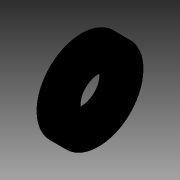
# Autodesk Inventor part: 2281_p2
Saved by Autodesk Inventor 2014 SP2 (Build 180246200, 246)
## iProperties
Created: 2019-11-08
Part Number: 2281_p2
Material: Generic
Catalog Web Link: www.cadenas.de
Description: 2281, 2282, 2280, 2290_p2-Roller Wheels
Vendor: 8020
Document SubType Name: Modeling
Designer: psadmin
Manufacturer: 8020
Mass: 0.492643 g
Surface Area: 5.37288 cm^2
Volume: 0.492643 cm^3
Density: 1 g/cm^3
Appearance: PSOLRGB-0-0-0
Category: PARTsolutions
Company: 8020
Title: 2281_p2
Author: Cadenas PARTsolutions
Comments: Roller Wheels
PSOL_IDENT_0: {$CADENAS_DATA\23d-libs\8020\inch\linear_motion\2281_p2.prj},178 {VTYP=3D},{NB=2281_p2},{LINA=2281_p
PSOL_IDENT_1: 2},{NN=2281, 2282, 2280, 2290_p2},{DATE=01.10.2019 06:04:24},{GEOMDATE=20.12.2011 00:00:00},{VERSION=
PSOL_IDENT_2: },{LINEID=10},{WBVAR=BT,RI},{WBNUMERIC=}  {NB=2281_p2},{LINA=2281_p2},{KT=DUMMY},{PN=2281},{NO=1},{M
PSOL_IDENT_3: AT=Self-lubricating, fiberglass-reinforced black nylon.},{BT=2},{BT1= '2','Permanent Lubricated Bron
PSOL_IDENT_4: ze Bushing' },{MT=10 Series},{RI=10},{RI1= '10','10 Series','15','15 Series' },{A=1.500},{B=1.125},{
PSOL_IDENT_5: C=0.240},{D=0.480},{E=0.563},{F=0.188},{G=0.314},{H=0.214},{J=0.118},{K=0.622},{L=0.429},{M=0.320},{
PSOL_IDENT_6: N=1/4-20},{N1=0.2500},{P=0.060},{Q=0.378},{W=.070},{G1=0.375},{K1=0.000}
NN: 2281, 2282, 2280, 2290_p2
NT: Roller Wheels
NB: 2281_p2
NBSYN: $PN._p2
LINA: 2281_p2
PN: 2281
MAT: Self-lubricating, fiberglass-reinforced black nylon.
BT: Permanent Lubricated Bronze Bushing
MT: 10 Series
RI: 10 Series
A: 1.5
B: 1.125
C: 0.24
D: 0.48
E: 0.563
F: 0.188
G: 0.314
H: 0.214
J: 0.118
K: 0.622
L: 0.429
M: 0.32
N: 1/4-20
P: 0.06
Q: 0.378
W: .070
SUPPLIER: 8020
ARTICLENO: 2281_p2
BOMINFO: 2281_p2
CREATOR: CADENAS GmbH
Autodesk Inventor part; units mm, degrees
ref_plane "YZ Plane" through (0, 0, 0) normal (1, 0, 0) x (0, 1, 0)
ref_plane "XZ Plane" through (0, 0, 0) normal (0, 1, 0) x (-1, 0, 0)
ref_plane "XY Plane" through (0, 0, 0) normal (0, 0, 1) x (1, 0, 0)
sketch "Sketch_1" plane through (0, 0, 0) normal (0, 0, 1) x (1, 0, 0)
  line L0 (1.4986, 0) -> (-1.4986, 0)
  line L1 (-1.4986, 3.175) -> (1.4986, 3.175)
  line L2 (1.4986, 3.175) -> (1.4986, 7.8994)
  line L3 (1.4986, 7.8994) -> (-1.4986, 7.8994)
  line L4 (-1.4986, 7.8994) -> (-1.4986, 3.175)
  constraints: 10 end point
revolve "Revolution1" add sketch "Sketch_1" angle 360 about axis through (1.4986, 0, 0) along (1, 0, 0)
ref_plane "P2_XY" through (-1.4986, 0, 0) normal (1, 0, 0) x (0, 0, -1)
ref_plane "P2_YZ" through (-1.4986, 0, 0) normal (0, 0, -1) x (0, 1, 0)
ref_plane "P2_ZX" through (-1.4986, 0, 0) normal (0, 1, 0) x (1, 0, 0)
body "Solid1"
